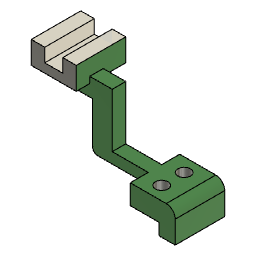
Figure-9 (Autodesk Fusion 360 design; units mm, degrees)
Autodesk Fusion 360 part; units mm, degrees
sketch "Sketch1" plane through (0, 0, 0) normal (0, 1, 0) x (1, 0, 0)
  line L0 (-18, 25) -> (0, 25)
  line L1 (-50.0002, -10) -> (-50, 12)
  line L2 (-50, 12) -> (-18, 12)
  line L3 (-18, 12) -> (-18, 25)
  line L4 (-50.0002, -10) -> (-10, -10)
  line L5 (0, 0) -> (0, 25)
  arc A0 (-10, -10) -> (0, 0) centre (-10, 0) ccw
  dimension "d6" = 18
  dimension "d7" = 50
  dimension "d8" = 13
  dimension "d10" = 22
  dimension "d11" = 10
  constraint perpendicular L0 L5
  constraint tangent L4 A0
  constraint tangent L5 A0
  measures "d6" distance of L0.start L0.end
  measures "d7" horizontal distance of L0.end L1.end
  measures "d8" distance of L0.start L2.end
  measures "d10" distance of L1.start L1.end
  measures "d11" radius of A0
extrude "Extrude1" add sketch "Sketch1" along normal mid plane 55
sketch "Sketch2" plane through (0, 0, 10) normal (0, 0, 1) x (-1, 0, 0)
  line L0 (10, 27.5) -> (10, -27.5)
  line L1 (10, -27.5) -> (50.0002, -27.5)
  line L2 (50.0002, -27.5) -> (50.0002, 27.5)
  line L3 (50.0002, 27.5) -> (10, 27.5)
  circle A0 centre (30.0002, 12.5) radius 7
  circle A1 centre (30.0002, -12.5) radius 7
  dimension "d17" = 14
  dimension "d18" = 15
  dimension "d19" = 20
  dimension "d20" = 14
  dimension "d21" = 15
  dimension "d22" = 20
  measures "d17" diameter of A0
  measures "d18" distance of L3 A0.centre
  measures "d19" distance of L2 A0.centre
  measures "d20" diameter of A1
  measures "d21" distance of L1 A1.centre
  measures "d22" distance of L2 A1.centre
extrude "Extrude2" cut sketch "Sketch2" against normal through all contours A0 | A1
sketch "Sketch3" plane through (0, 0, 0) normal (0, 1, 0) x (1, 0, 0)
  line L0 (-50, 2) -> (-112, 2)
  line L1 (-50, -10) -> (-90, -10)
  line L2 (-112, 2) -> (-112, -50)
  line L3 (-90, -10) -> (-90, -70)
  line L4 (-90, -70) -> (-165, -70)
  line L5 (-165, -70) -> (-165, -50)
  line L6 (-165, -50) -> (-112, -50)
  line L7 (-50, -10) -> (-50, 2)
  dimension "d24" = 62
  dimension "d26" = 40
  dimension "d28" = 52
  dimension "d30" = 75
  dimension "d31" = 20
  dimension "d52" = 12
  constraint horizontal L0
  constraint horizontal L1
  constraint perpendicular L0 L2
  constraint perpendicular L1 L3
  constraint perpendicular L3 L4
  constraint perpendicular L4 L5
  constraint perpendicular L2 L6
  constraint perpendicular L0 L7
  measures "d24" distance of L0.start L0.end
  measures "d26" distance of L1.start L1.end
  measures "d28" distance of L0.end L2.end
  measures "d30" distance of L3.end L4.end
  measures "d31" distance of L4.end L5.end
  measures "d52" vertical distance of L0.end L1.end
extrude "Extrude3" add sketch "Sketch3" along normal mid plane 15
fillet "Fillet1" radius 6 1 edges at (-112, 0, -2)
sketch "Sketch5" plane through (0, -7.5, 0) normal (0, -1, 0) x (1, 0, 0)
  arc A0 (-112, 4) -> (-106, -2) centre (-106, 4) ccw
  line L0 (-106, -2) -> (-50.0001, -2)
  line L1 (-50.0001, -2) -> (-50.0002, 10)
  line L2 (-50.0002, 10) -> (-90, 10)
  line L3 (-90, 10) -> (-90, 70)
  line L4 (-90, 70) -> (-165, 70)
  line L5 (-165, 70) -> (-165, 50)
  line L6 (-165, 50) -> (-112, 50)
  line L7 (-112, 50) -> (-112, 4)
  line L8 (-115, 63) -> (-165, 63)
  line L9 (-165, 63) -> (-165, 88)
  line L10 (-165, 88) -> (-150, 88)
  line L11 (-150, 88) -> (-150, 73)
  line L12 (-150, 73) -> (-130, 73)
  line L13 (-130, 73) -> (-130, 88)
  line L14 (-130, 88) -> (-115, 88)
  line L15 (-115, 88) -> (-115, 63)
  dimension "d41" = 50
  dimension "d42" = 25
  dimension "d43" = 15
  dimension "d44" = 15
  dimension "d45" = 20
  dimension "d46" = 15
  dimension "d47" = 18
  constraint parallel L4 L8
  constraint perpendicular L8 L9
  constraint perpendicular L9 L10
  constraint perpendicular L10 L11
  constraint perpendicular L11 L12
  constraint perpendicular L10 L13
  constraint perpendicular L13 L14
  constraint perpendicular L8 L15
  constraint collinear L5 L9
  measures "d41" distance of L8.start L8.end
  measures "d42" distance of L8.end L9.end
  measures "d43" distance of L10.end L11.end
  measures "d44" distance of L9.end L10.end
  measures "d45" distance of L11.end L12.end
  measures "d46" distance of L12.end L13.end
  measures "d47" vertical distance of L3.end L14.end
extrude "Extrude4" add sketch "Sketch5" along normal blind 15 and the other way blind 40 contours L4 L5 L8 L9 L15 | L4 L9 L10 L11 L12 L13 L14 L15
sketch "Sketch6" plane through (0, -7.5, 0) normal (0, -1, 0) x (1, 0, 0)
  line L0 (-115, 63) -> (-165, 63)
  line L1 (-165, 63) -> (-165, 50)
  line L2 (-165, 50) -> (-112, 50)
  line L3 (-112, 50) -> (-112, 4)
  arc A0 (-112, 4) -> (-106, -2) centre (-106, 4) ccw
  line L4 (-106, -2) -> (-50.0001, -2)
  line L5 (-50.0001, -2) -> (-50.0002, 10)
  line L6 (-50.0002, 10) -> (-90, 10)
  line L7 (-90, 10) -> (-90, 70)
  line L8 (-90, 70) -> (-115, 70)
  line L9 (-115, 70) -> (-115, 63)
sketch "Sketch7" plane through (0, -7.5, 0) normal (0, -1, 0) x (1, 0, 0)
